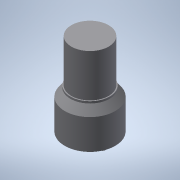
# Autodesk Inventor part: moter
Saved by Autodesk Inventor 2020 (Build 240168000, 168)
## iProperties
Created: 2017-11-27
Part Number: moter
Material: 一般
Document SubType Name: Modeling
Designer: USER
Density: 1 g/cm^3
Appearance: Default
Author: USER
Autodesk Inventor part; units mm, degrees
ref_plane "YZ Plane" through (0, 0, 0) normal (1, 0, 0) x (0, 1, 0)
ref_plane "XZ Plane" through (0, 0, 0) normal (0, 1, 0) x (-1, 0, 0)
ref_plane "XY Plane" through (0, 0, 0) normal (0, 0, 1) x (1, 0, 0)
sketch "草圖1" plane through (0, 0, 0) normal (0, 0, 1) x (1, 0, 0)
  circle A0 centre (0, 0) radius 12.85
  dimension "d0" = 25.7
  constraints: 1 centre point, 1 coincident
  measures "d0" diameter of A0
extrude "擠出1" add sketch "草圖1" along normal blind 26
sketch "草圖2" plane through (0, 0, 26) normal (0, 0, 1) x (1, 0, 0)
  circle A0 centre (0, 0) radius 10
  circle A1 centre (0, 0) radius 12.85 projected
  dimension "d3" = 20
  constraints: 1 centre point, 1 coincident
  measures "d3" diameter of A0
extrude "擠出2" cut sketch "草圖2" against normal blind 1
sketch "草圖3" plane through (0, 0, 0) normal (0, 1, 0) x (-1, 0, 0)
  line L0 (-12.85, 25) -> (12.85, 25) projected
  line L1 (10, 26) -> (10, 25) projected
  line L2 (10, 25) -> (12.85, 21)
  line L3 (12.85, 0) -> (12.85, 25) projected
  line L4 (0, -5.2) -> (0, 31.2) projected
  point P0 (0, 0)
  dimension "d6" = 4
  constraints: 2 end point, 1 point on line
  measures "d6" distance from line of L0 L2.end
revolve "迴轉1" cut sketch "草圖3" angle 360 about axis through (0, 0, -10) along (0, 0, 1)
sketch "草圖4" plane through (0, 0, 0) normal (0, 0, -1) x (-1, 0, 0)
  circle A0 centre (0, 0) radius 5
  circle A1 centre (0, 0) radius 12.85 projected
  dimension "d8" = 10
  constraints: 1 centre point, 1 coincident
  measures "d8" diameter of A0
extrude "擠出3" cut sketch "草圖4" against normal blind 2
sketch "草圖5" plane through (0, 0, 2) normal (0, 0, -1) x (-1, 0, 0)
  circle A0 centre (0, 0) radius 10.5
  circle A1 centre (0, 0) radius 12.85 projected
  dimension "d11" = 21
  constraints: 1 centre point, 1 coincident
  measures "d11" diameter of A0
extrude "擠出4" cut sketch "草圖5" against normal blind 3
sketch "草圖6" plane through (0, 0, 2) normal (0, 0, -1) x (-1, 0, 0)
  line L0 (0, 0) -> (-13.3502, 0) construction
  line L1 (0, 0) -> (8.2303, -14.2554) construction
  line L2 (0, 0) -> (8.5219, 14.7603) construction
  line L3 (-10.3078, -2) -> (-4.5826, -2)
  line L4 (-10.3078, 2) -> (-4.5826, 2)
  circle A0 centre (0, 0) radius 5 projected
  circle A1 centre (0, 0) radius 10.5 projected
  line L5 (0.5592, -4.9686) -> (3.4218, -9.9268)
  line L6 (4.0233, -2.9686) -> (6.8859, -7.9268)
  line L7 (4.0233, 2.9686) -> (6.8859, 7.9268)
  line L8 (0.5592, 4.9686) -> (3.4218, 9.9268)
  dimension "d14" = 120
  dimension "d15" = 120
  dimension "d16" = 2
  dimension "d17" = 2
  dimension "d18" = 4
  dimension "d19" = 2
  dimension "d20" = 2
  dimension "d21" = 2
  constraints: 18 end point, 12 point on circle, 5 parallel, 2 horizontal
  measures "d14" angle of L1 L2
  measures "d15" angle of L0 L2
  measures "d16" distance between parallel lines of L0 L4
  measures "d17" distance between parallel lines of L3 L0
  measures "d18" distance between parallel lines of L7 L8
  measures "d19" distance between parallel lines of L2 L8
  measures "d20" distance between parallel lines of L1 L6
  measures "d21" distance between parallel lines of L1 L5
extrude "擠出5" cut sketch "草圖6" against normal blind 10 contours L3 A0 L5 A1 | A1 L8 A0 L4 | L6 A0 L7 A1
fillet "圓角1" radius 3 3 edges at (10.5, 0, 2) (-5.25, 9.0933, 2) (-5.25, -9.0933, 2)
sketch "草圖8" plane through (0, 0, 0) normal (0, 1, 0) x (-1, 0, 0)
  line L0 (-12.85, 5) -> (-12.85, 5.6297)
  line L1 (0, -5.2) -> (0, 31.2) projected
  line L2 (-12.85, 5.6297) -> (-10.5, 5)
  line L3 (12.85, 5) -> (-12.85, 5) projected
  line L4 (-10.5, 5) -> (-10.3078, 5) projected
  point P0 (0, 0)
  dimension "d28" = 15
  constraints: 4 end point, 1 vertical
  measures "d28" angle of L3 L2
revolve "迴轉2" cut sketch "草圖8" angle 360 about axis through (0, 0, -10) along (0, 0, 1)
sketch "草圖9" plane through (0, 0, 26) normal (0, 0, 1) x (1, 0, 0)
  circle A0 centre (0, 0) radius 9.5
  dimension "d29" = 19
  constraints: 1 centre point, 1 coincident
  measures "d29" diameter of A0
extrude "擠出6" add sketch "草圖9" along normal blind 21.787
equation "\"d15\" = d14"
equation "\"d17\" = d16"
equation "\"d20\" = d19"
equation "\"d21\" = d19"
